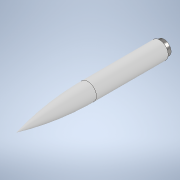
# Autodesk Inventor part: nose cone n2
Saved by Autodesk Inventor 2020 (Build 240168000, 168)
## iProperties
Created: 2022-02-04
Part Number: nose cone n2
Material: Generic
Document SubType Name: Modeling
Designer: User
Density: 1 g/cm^3
Appearance: Semi-Polished
Author: User
Autodesk Inventor part; units mm, degrees
ref_plane "YZ Plane" through (0, 0, 0) normal (1, 0, 0) x (0, 1, 0)
ref_plane "XZ Plane" through (0, 0, 0) normal (0, 1, 0) x (-1, 0, 0)
ref_plane "XY Plane" through (0, 0, 0) normal (0, 0, 1) x (1, 0, 0)
sketch "Sketch1" plane through (0, 0, 0) normal (1, 0, 0) x (0, 1, 0)
  line L0 (-46.288, 11.5067) -> (-46.288, -488.4933) construction
  line L1 (-46.288, 11.5067) -> (-46.288, -488.4933)
  line L2 (-46.288, -488.4933) -> (-76.288, -488.4933)
  line L3 (-76.288, -488.4933) -> (-76.288, -238.4933)
  arc A0 (-46.288, 11.5067) -> (-76.288, -238.4933) centre (980.3786, -238.4933) ccw
  arc A1 (-46.288, -238.4933) -> (-46.288, 11.5067) centre (-2732.9697, -113.4933) ccw construction
  line L4 (-71.288, -488.4933) -> (-71.288, -503.4933)
  line L5 (-71.288, -503.4933) -> (-46.288, -503.4933)
  line L6 (-46.288, -488.4933) -> (-46.288, -503.4933)
  point P0 (0, 0)
  dimension "d0" = 500
  dimension "d1" = 500
  dimension "d2" = 250
  dimension "d3" = 30
  dimension "d4" = 30
  dimension "d6" = 15
  dimension "d7" = 25
  constraints: 14 end point, 5 point on circle, 4 vertical, 2 centre point, 2 perpendicular, 1 horizontal, 1 midpoint, 1 point on line, 1 tangent
  measures "d0" distance of L0.start L0.end
  measures "d1" distance of L1.start L1.end
  measures "d2" distance of L2.end L3.end
  measures "d3" distance between parallel lines of L3 L0
  measures "d4" distance between parallel lines of L3 L1
  measures "d6" distance of L4.start L4.end
  measures "d7" distance of L4.end L5.end
revolve "Revolution1" add sketch "Sketch1" angle 360 about axis through (0, -46.288, 11.5067) along (0, 0, -1)
body "Solid1"
